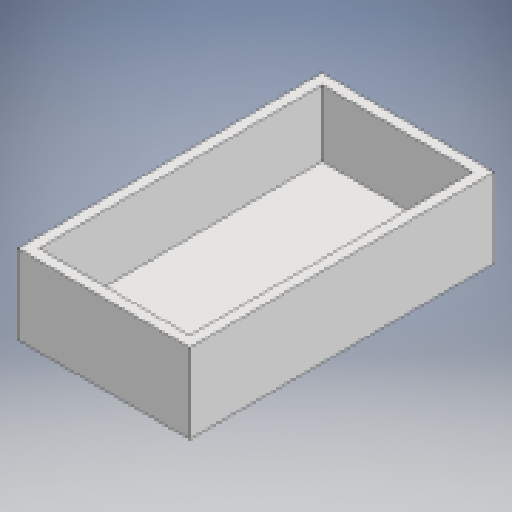
# Autodesk Inventor part: gps_case_2
Saved by Autodesk Inventor 2025.2 (Build 292293000, 293)
## iProperties
Created: 2024-02-08
Part Number: gps_case_2
Material: 일반
Document SubType Name: Modeling
Designer: ps737
Density: 1 g/cm^3
Appearance: 기본값
Author: ps737
Autodesk Inventor part; units mm, degrees
ref_plane "YZ Plane" through (0, 0, 0) normal (1, 0, 0) x (0, 1, 0)
ref_plane "XZ Plane" through (0, 0, 0) normal (0, 1, 0) x (-1, 0, 0)
ref_plane "XY Plane" through (0, 0, 0) normal (0, 0, 1) x (1, 0, 0)
sketch "스케치2" plane through (0, 0, 0) normal (0, 1, 0) x (-1, 0, 0)
  line L0 (65, -2.8774) -> (0, -2.8774)
  line L1 (0, -2.8774) -> (0, -117.8774)
  line L2 (0, -117.8774) -> (65, -117.8774)
  line L3 (65, -117.8774) -> (65, -2.8774)
  line L4 (61, -6.8774) -> (4, -6.8774)
  line L5 (4, -6.8774) -> (4, -113.8774)
  line L6 (4, -113.8774) -> (61, -113.8774)
  line L7 (61, -113.8774) -> (61, -6.8774)
  point P0 (0, 0)
  dimension "d0" = 65
  dimension "d1" = 115
  dimension "d2" = 4
  constraints: 16 end point, 4 parallel, 2 perpendicular, 1 horizontal, 3 other
  measures "d0" distance between parallel lines of L1 L3
  measures "d1" distance between parallel lines of L2 L0
  measures "d2" distance between parallel lines of L3 L7
extrude "돌출1" add sketch "스케치2" along normal blind 30
extrude "돌출2" add sketch "스케치2" along normal blind 5 contours L7 L6 L5 L4
